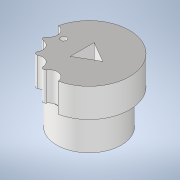
# Autodesk Inventor part: handle_base2
Saved by Autodesk Inventor 2021 (Build 250183000, 183)
## iProperties
Created: 2021-06-02
Part Number: handle_base2
Material: Generic
Document SubType Name: Modeling
Designer: teh18
Density: 1 g/cm^3
Appearance: Default
Author: teh18
Autodesk Inventor part; units mm, degrees
ref_plane "YZ Plane" through (0, 0, 0) normal (1, 0, 0) x (0, 1, 0)
ref_plane "XZ Plane" through (0, 0, 0) normal (0, 1, 0) x (-1, 0, 0)
ref_plane "XY Plane" through (0, 0, 0) normal (0, 0, 1) x (1, 0, 0)
sketch "Sketch1" plane through (0, 0, 0) normal (0, 0, 1) x (1, 0, 0)
  line L0 (-6, 0) -> (-6, 10.3923) projected
  line L1 (-6, 10.3923) -> (3, 5.1962) projected
  line L2 (3, 5.1962) -> (12, 0) projected
  line L3 (12, 0) -> (3, -5.1962) projected
  line L4 (3, -5.1962) -> (-6, -10.3923) projected
  line L5 (-6, -10.3923) -> (-6, 0) projected
  circle A0 centre (0, 0) radius 27.5 projected
  circle A1 centre (0, 0) radius 35
  circle A2 centre (-35, 0) radius 7.5
  circle A3 centre (-30.3109, 17.5) radius 7.5
  circle A4 centre (-17.5, 30.3109) radius 7.5
  circle A5 centre (0, 35) radius 7.5
  point P0 (0, 27.5)
  point P1 (-7.4568, 34.1964)
  point P2 (-10.6404, 33.3434)
  point P3 (-13.75, 23.8157)
  point P4 (7.4568, 34.1964)
  point P5 (-27.5, 0)
  point P6 (-34.1964, -7.4568)
  point P7 (-23.556, 25.8866)
  point P8 (-25.8866, 23.556)
  point P9 (-23.8157, 13.75)
  point P10 (-33.3434, 10.6404)
  point P11 (-34.1964, 7.4568)
  dimension "d5" = 70
  dimension "d8" = 90
  constraints: 4 centre point, 1 coincident, 1 tangent, 10 other
ref_plane "Work Plane1" through (-28, -28, 55) normal (0, 0, -1) x (0, 1, 0)
ref_plane "Work Plane2" through (-38, -38, 45) normal (0, 0, -1) x (0, 1, 0)
ref_plane "Work Plane4" through (-38, -38, 25) normal (0, 0, -1) x (0, 1, 0)
extrude "Extrusion1" add sketch "Sketch1" along normal up to surface (25 mm away) contours A0 | A2 A1 A3 A0 | A0 A5 A1 A2 | A3 A1 A4 A0 | A0 A4 A1 A5
ref_plane "Work Plane5" through (-80, -43, 35) normal (0, 0, -1) x (0, 1, 0)
fillet "Fillet1" radius 2 6 edges at (-7.4568, 34.1964, 12.5) (-10.6404, 33.3434, 12.5) (-23.556, 25.8866, 12.5) (-25.8866, 23.556, 12.5) (-33.3434, 10.6404, 12.5) (-34.1964, 7.4568, 12.5)
sketch "Sketch3" plane through (0, 0, 25) normal (0, 0, 1) x (0.7071068, -0.7071068, 0)
  circle A0 centre (0, 0) radius 28 projected
  point P0 (0, 0)
ref_plane "Work Plane3" through (-80, -43, 55) normal (0, 0, -1) x (0, 1, 0)
extrude "Extrusion3" add sketch "Sketch3" along normal blind 10
body "Solid1"
